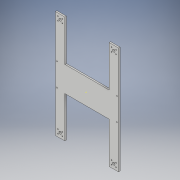
# Autodesk Inventor part: chassis mit motorlöcher
Saved by Autodesk Inventor 2018 (Build 220112000, 112)
## iProperties
Created: 2018-01-20
Part Number: chassis mit motorlöcher
Material: Generisch
Document SubType Name: Modeling
Designer: fhinstall
Density: 1 g/cm^3
Appearance: Vorgabe
Author: fhinstall
Autodesk Inventor part; units mm, degrees
ref_plane "YZ Plane" through (0, 0, 0) normal (1, 0, 0) x (0, 1, 0)
ref_plane "XZ Plane" through (0, 0, 0) normal (0, 1, 0) x (-1, 0, 0)
ref_plane "XY Plane" through (0, 0, 0) normal (0, 0, 1) x (1, 0, 0)
sketch "Skizze1" plane through (0, 0, 0) normal (0, 1, 0) x (-1, 0, 0)
  line L0 (127.3199, 0) -> (-102.7808, 0) construction
  line L1 (0, 142.2638) -> (0, -235.5235) construction
  line L2 (100, 50) -> (100, 0)
  line L3 (70, 40) -> (0, 40)
  line L4 (0, 0) -> (100, 0)
  line L5 (0, 40) -> (0, 0)
  line L6 (100, 50) -> (100, 170)
  line L7 (100, 170) -> (70, 170)
  line L8 (70, 170) -> (70, 40)
  circle A0 centre (95, 36) radius 1.7
  line L9 (100, 140) -> (70, 140) construction
  circle A1 centre (85, 155) radius 4
  circle A2 centre (85, 155) radius 9.5 construction
  line L10 (92.1979, 148.8) -> (77.8021, 148.8) construction
  line L11 (77.8021, 148.8) -> (77.8021, 161.2) construction
  line L12 (77.8021, 161.2) -> (92.1979, 161.2) construction
  line L13 (92.1979, 161.2) -> (92.1979, 148.8) construction
  line L14 (92.1979, 148.8) -> (77.8021, 161.2) construction
  line L15 (77.8021, 148.8) -> (92.1979, 161.2) construction
  circle A3 centre (77.8021, 161.2) radius 1.7
  circle A4 centre (92.1979, 161.2) radius 1.7
  circle A5 centre (92.1979, 148.8) radius 1.7
  circle A6 centre (77.8021, 148.8) radius 1.7
  dimension "d62" = 19
  dimension "d10" = 100
  dimension "d12" = 30
  dimension "d13" = 170
  dimension "d14" = 40
  dimension "d22" = 5
  dimension "d23" = 4
  dimension "d26" = 3.4
  dimension "d59" = 30
  dimension "d60" = 8
  dimension "d61" = 15
  dimension "d63" = 12.4
  dimension "d64" = 3.4
  dimension "d65" = 3.4
  dimension "d66" = 3.4
  dimension "d67" = 3.4
  dimension "d69" = 8.8
  dimension "d70" = 7.8021
  constraints: 32 end point, 7 perpendicular, 6 centre point, 6 point on line, 5 coincident, 2 horizontal, 2 midpoint, 2 parallel, 2 vertical, 1 collinear, 3 other
  measures "d10" distance between parallel lines of L1 L2
  measures "d12" distance of L6.end L7.end
  measures "d13" distance between parallel lines of L0 L7
  measures "d14" distance between parallel lines of L0 L3
  measures "d22" distance from line of L2 A0.centre
  measures "d23" distance from line of L3 A0.centre
  measures "d26" diameter of A0
  measures "d59" distance between parallel lines of L9 L7
  measures "d60" diameter of A1
  measures "d61" distance from line of L9 A1.centre
  measures "d63" distance of L10.end L11.end
  measures "d64" diameter of A6
  measures "d65" diameter of A5
  measures "d66" diameter of A4
  measures "d67" diameter of A3
  measures "d69" distance from line of L7 L12.end
  measures "d70" distance from line of L6 A4.centre
extrude "Extrusion1" add sketch "Skizze1" along normal blind 5
ref_plane "Arbeitsebene1" through (0, 0, 40) normal (1, 0, 0) x (0, 1, 0)
ref_plane "Arbeitsebene2" through (0, 5, 0) normal (0, 0, -1) x (-1, 0, 0)
mirror "Spiegeln1" about plane through (0, 5, 0) normal (0, 0, -1) of "Extrusion1"
pattern_circular "Runde Anordnung1" count 2 over 360 about axis through (0, 5, 0) along (0, -1, 0) of "Extrusion1"
mirror "Spiegeln2" about plane through (0, 0, 40) normal (1, 0, 0) of "Extrusion1"
mirror "Spiegeln3" about plane through (0, 5, 0) normal (0, 0, -1) of "Extrusion1"
